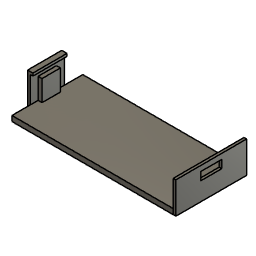
Teensy 4.1 Mount (Autodesk Fusion 360 design; units mm, degrees)
Autodesk Fusion 360 part; units mm, degrees
sketch "Sketch1" plane through (0, 0, 0) normal (0, 1, 0) x (1, 0, 0)
  line L0 (0, 27) -> (61.5, 27)
  line L1 (61.5, 27) -> (61.5, 0)
  line L2 (61.5, 0) -> (0, 0)
  line L3 (0, 0) -> (0, 27)
  dimension "d1" = 27
  dimension "d2" = 61.5
  constraint horizontal L0
  constraint vertical L1
  constraint horizontal L2
  constraint vertical L3
  constraint coincident L2.end L3.start
  measures "d1" distance of L0.end L1.end
  measures "d2" distance of L0.start L0.end
extrude "Extrude1" add sketch "Sketch1" along normal blind 2 makes body 1
sketch "Sketch2" plane through (61.5, 0, 0) normal (1, 0, 0) x (0, 0, -1)
  line L0 (0, 0) -> (27, 0)
  line L1 (27, 0) -> (27, 2)
  line L2 (27, 2) -> (0, 2)
  line L3 (0, 2) -> (0, 0)
  line L4 (0, 12) -> (27, 12)
  line L5 (27, 12) -> (27, 0)
  line L6 (27, 0) -> (0, 0)
  line L7 (0, 0) -> (0, 12)
  dimension "d5" = 10
  constraint horizontal L4
  constraint vertical L5
  constraint horizontal L6
  constraint vertical L7
  constraint coincident L0.start L3.end
  constraint coincident L0.end L1.start
  measures "d5" distance of L2 L4
extrude "Extrude2" add sketch "Sketch2" along normal blind 1 separate body makes body 2
sketch "Sketch3" plane through (62.5, 0, 0) normal (1, 0, 0) x (0, 0, -1)
  line L0 (0, 0) -> (27, 0)
  line L1 (27, 0) -> (27, 12)
  line L2 (27, 12) -> (0, 12)
  line L3 (0, 12) -> (0, 0)
  line L4 (9.5, 10) -> (17.5, 10)
  line L5 (17.5, 10) -> (17.5, 6.94)
  line L6 (17.5, 6.94) -> (9.5, 6.94)
  line L7 (9.5, 6.94) -> (9.5, 10)
  line L8 (13.5, 12) -> (13.5, 0) construction
  point P0 (13.5, 6.94)
  dimension "d8" = 8
  dimension "d9" = 3.06
  dimension "d10" = 2
  constraint horizontal L4
  constraint vertical L5
  constraint horizontal L6
  constraint vertical L7
  constraint midpoint L2 L8.start
  constraint midpoint L0 L8.end
  constraint midpoint L6 P0
  constraint coincident L8 P0
  measures "d8" distance of L4.start L4.end
  measures "d9" distance of L4.end L5.end
  measures "d10" distance of L2 L4
extrude "Extrude3" cut sketch "Sketch3" against normal up to surface (1 mm away) contours L4 L5 L6 L7 bodies 2
sketch "Sketch5" plane through (0, 0, 0) normal (-1, 0, 0) x (0, 0, 1)
  line L0 (-27, 0) -> (0, 0)
  line L1 (0, 0) -> (0, 2)
  line L2 (0, 2) -> (-27, 2)
  line L3 (-27, 2) -> (-27, 0)
  line L4 (-20, 12) -> (-7, 12)
  line L5 (-7, 12) -> (-7, 0)
  line L6 (-7, 0) -> (-20, 0)
  line L7 (-20, 0) -> (-20, 12)
  line L8 (0, 12) -> (-27, 12) construction
  point P0 (-13.5, 0)
  dimension "d15" = 13
  constraint horizontal L4
  constraint vertical L5
  constraint horizontal L6
  constraint vertical L7
  constraint coincident L0 L5.end
  constraint midpoint L0 P0
  constraint midpoint L6 P0
  constraint coincident L4.end L8
  measures "d15" distance of L4.start L4.end
extrude "Extrude5" add sketch "Sketch5" along normal blind 1 contours L0 L2 L5 L6 L7 | L2 L4 L5 L7 bodies 1
sketch "Sketch6" plane through (0, 12, 0) normal (0, 1, 0) x (-1, 0, 0)
  line L0 (0, -7) -> (0, -20)
  line L1 (0, -20) -> (1, -20)
  line L2 (1, -20) -> (1, -7)
  line L3 (1, -7) -> (0, -7)
  line L4 (1, -20) -> (-1, -20)
  line L5 (-1, -20) -> (-1, -7)
  line L6 (-1, -7) -> (1, -7)
  line L7 (1, -7) -> (1, -20)
  dimension "d19" = 1
  constraint horizontal L4
  constraint vertical L5
  constraint horizontal L6
  constraint vertical L7
  constraint coincident L2.end L3.start
  constraint coincident L1.end L2.start
  measures "d19" distance of L0 L5
extrude "Extrude6" add sketch "Sketch6" along normal blind 1 bodies 1
sketch "Sketch7" plane through (0, 0, 0) normal (1, 0, 0) x (0, 0, -1)
  line L0 (7, 2) -> (20, 2)
  line L1 (20, 2) -> (20, 12)
  line L2 (20, 12) -> (7, 12)
  line L3 (7, 12) -> (7, 2)
  line L4 (10, 9.95) -> (17, 9.95)
  line L5 (17, 9.95) -> (17, 2)
  line L6 (17, 2) -> (10, 2)
  line L7 (10, 2) -> (10, 9.95)
  point P0 (13.5, 2)
  dimension "d22" = 2.05
  dimension "d23" = 7
  constraint horizontal L4
  constraint vertical L5
  constraint horizontal L6
  constraint vertical L7
  constraint midpoint L6 P0
  constraint midpoint L0 P0
  measures "d22" distance of L2 L4
  measures "d23" distance of L4.start L4.end
extrude "Extrude7" add sketch "Sketch7" along normal blind 1.5 contours L0 L4 L5 L6 L7 bodies 1
